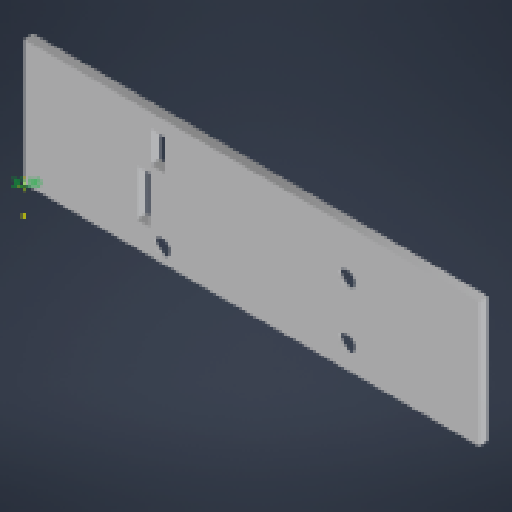
# Autodesk Inventor part: Tyl
Saved by Autodesk Inventor 2023 (Build 270158000, 158)
## iProperties
Created: 2022-02-03
Part Number: Tyl
Material: Aluminium 6061
Document SubType Name: Modeling
Designer: Michał
Density: 2.7 g/cm^3
Appearance: Aluminium — płaski
Mass: 15.0029 g
Surface Area: 61.813 cm^2
Volume: 5.55662 cm^3
Author: Michał
Autodesk Inventor part; units mm, degrees
ref_plane "YZ Plane" through (0, 0, 0) normal (1, 0, 0) x (0, 1, 0)
ref_plane "XZ Plane" through (0, 0, 0) normal (0, 1, 0) x (-1, 0, 0)
ref_plane "XY Plane" through (0, 0, 0) normal (0, 0, 1) x (1, 0, 0)
sketch "Szkic1" plane through (0, 0, 0) normal (1, 0, 0) x (0, 1, 0)
  line L0 (6, 0) -> (6, -2)
  line L1 (6, -2) -> (33, -2)
  line L2 (33, -2) -> (33, 0)
  line L3 (33, 0) -> (6, 0)
  line L4 (31, 0) -> (31, 2.3) construction
  line L5 (6, 0) -> (31, 0) construction
  line L6 (6, 5) -> (6, 0) construction
  dimension "d1" = 2
  dimension "d27" = 2
  constraints: 8 end point, 3 perpendicular, 2 collinear, 1 vertical
  measures "d1" distance between parallel lines of L3 L1
  measures "d27" distance between parallel lines of L2 L4
extrude "Wyciągnięcie proste1" add sketch "Szkic1" along normal blind 98
sketch "Szkic2" plane through (0, 6, -2) normal (0, 0, -1) x (-1, 0, 0)
  circle A0 centre (-69.5896, 17) radius 1.2295 construction
  circle A1 centre (-69.5896, 5) radius 1.2295 construction
  circle A2 centre (-29.7896, 3) radius 1.2295 construction
  constraints: 3 coincident
hole "Otwór1" at (69.5896, 23, -2) at (69.5896, 11, -2) at (29.7896, 9, -2) direction (0, 0, 1) diameter 3.4 depth 5.5 tip angle 118 countersink diameter 6.9 countersink angle 84.225 clearance for "Śruba ze łbem stożkowym ISO 2009/7046" size "M3" standard "ISO"
sketch "Szkic3" plane through (0, 6, -2) normal (0, 0, -1) x (-1, 0, 0)
  line L0 (-32.2896, 0) -> (-32.2896, 25) projected
  line L1 (-27.0896, 5.55) -> (-24.3896, 5.55)
  line L2 (-24.3896, 5.55) -> (-24.3896, 15.55)
  line L3 (-24.3896, 15.55) -> (-27.0896, 15.55)
  line L4 (-27.0896, 15.55) -> (-27.0896, 5.55)
  line L5 (-30.2896, 23.9) -> (-27.2896, 23.9)
  line L6 (-27.2896, 23.9) -> (-27.2896, 17.2)
  line L7 (-27.2896, 17.2) -> (-30.2896, 17.2)
  line L8 (-30.2896, 17.2) -> (-30.2896, 23.9)
  point P0 (0, -6)
  dimension "d17" = 5.2
  dimension "d18" = 5.55
  dimension "d19" = 2.7
  dimension "d20" = 10
  dimension "d21" = 2
  dimension "d22" = 17.2
  dimension "d23" = 6.7
  dimension "d24" = 3
  constraints: 16 end point, 4 parallel, 2 horizontal, 2 perpendicular
  measures "d17" distance between parallel lines of L0 L4
  measures "d18" distance from line of L0.start L1
  measures "d19" distance between parallel lines of L2 L4
  measures "d20" distance of L1.end L2.end
  measures "d21" distance between parallel lines of L0 L8
  measures "d22" distance from line of L0.start L7
  measures "d23" distance of L5.end L6.end
  measures "d24" distance of L5.start L5.end
extrude "Wyciągnięcie proste2" cut sketch "Szkic3" against normal up to next
sketch "Sketch4" plane through (0, 0, 0) normal (-1, 0, 0) x (0, 0, 1)
  line L0 (-2, 6) -> (-2, 33) construction
  line L1 (-2, 6) -> (-2, 7.1547)
  line L2 (0, 6) -> (-2, 6)
  line L3 (-2, 7.1547) -> (0, 6)
  point P0 (0, 0)
  dimension "d31" = 30
  constraints: 6 end point, 1 perpendicular, 1 point on line
  measures "d31" angle of L3 L2
extrude "Extrusion3" cut sketch "Sketch4" against normal through all
